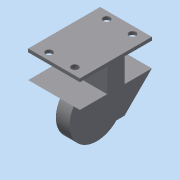
# Autodesk Inventor part: caster wheel
Saved by Autodesk Inventor 2015 (Build 190159000, 159)
## iProperties
Created: 2015-06-24
Part Number: caster wheel
Material: Generic
Document SubType Name: Modeling
Designer: Rahul
Density: 1 g/cm^3
Appearance: Default
Author: Rahul
Autodesk Inventor part; units mm, degrees
ref_plane "YZ Plane" through (0, 0, 0) normal (1, 0, 0) x (0, 1, 0)
ref_plane "XZ Plane" through (0, 0, 0) normal (0, 1, 0) x (-1, 0, 0)
ref_plane "XY Plane" through (0, 0, 0) normal (0, 0, 1) x (1, 0, 0)
sketch "Sketch10" plane through (0, 0, 0) normal (0, 1, 0) x (-1, 0, 0)
  line L0 (24.0538, -33.4645) -> (-24.0538, -33.4645)
  line L1 (-24.0538, -33.4645) -> (-24.0538, 33.4645)
  line L2 (-24.0538, 33.4645) -> (24.0538, 33.4645)
  line L3 (24.0538, 33.4645) -> (24.0538, -33.4645)
  line L4 (33.6753, 0) -> (-33.6753, 0) projected
  line L5 (0, -46.8503) -> (0, 46.8503) projected
  point P0 (0, 0)
  dimension "d17" = 66.929
  dimension "d18" = 48.1076
  constraints: 8 end point, 2 parallel, 1 horizontal, 1 perpendicular, 2 other
  measures "d17" distance of L0.end L1.end
  measures "d18" distance of L0.start L0.end
extrude "Extrusion4" add sketch "Sketch10" against normal blind 50.8
sketch "Sketch11" plane through (0, -50.8, 0) normal (0, -1, 0) x (1, 0, 0)
  line L0 (6.35, 25.4) -> (-6.35, 25.4)
  line L1 (-6.35, 25.4) -> (-6.35, 0)
  line L2 (-6.35, 0) -> (6.35, 0)
  line L3 (6.35, 0) -> (6.35, 25.4)
  line L4 (-33.6753, 0) -> (33.6753, 0) projected
  line L5 (0, -46.8503) -> (0, 46.8503) projected
  point P0 (0, 0)
  dimension "d21" = 25.4
  dimension "d22" = 12.7
  constraints: 8 end point, 2 parallel, 1 collinear, 1 horizontal, 1 perpendicular, 1 other
  measures "d21" distance of L2.end L0.start
  measures "d22" distance of L1.end L2.end
revolve "Revolution3" add sketch "Sketch11" angle 360 about axis through (-6.35, -50.8, 0) along (1, 0, 0)
chamfer "Chamfer2" distance 25.4 angle 45 2 edges at (0, -50.8, -33.4645) (0, -50.8, 33.4645)
sketch "Sketch12" plane through (0, 0, 0) normal (0, 1, 0) x (1, 0, 0)
  circle A0 centre (12.7508, 26.7462) radius 3.2195
  line L0 (-24.0538, 33.4645) -> (24.0538, 33.4645) projected
  line L1 (24.0538, 33.4645) -> (24.0538, 8.0645) projected
  circle A1 centre (-11.2649, 26.7462) radius 3.2195
  circle A2 centre (12.7508, -26.8097) radius 3.2195
  circle A3 centre (-11.2649, -26.8097) radius 3.2195
  point P0 (0, 0)
  dimension "d27" = 6.4389
  dimension "d28" = 6.7183
  dimension "d29" = 11.303
  dimension "d32" = 24.0157
  dimension "d42" = 53.5559
  dimension "d46" = 24.0157
  constraints: 4 centre point, 2 horizontal, 1 vertical, 6 other
  measures "d27" diameter of A0
  measures "d28" distance from line of L0 A0.centre
  measures "d29" distance from line of L1 A0.centre
  measures "d32" distance of A0.centre A1.centre
  measures "d42" distance of A0.centre A2.centre
  measures "d46" distance of A2.centre A3.centre
extrude "Extrusion5" cut sketch "Sketch12" against normal blind 5.08
sketch "Sketch13" plane through (-24.0538, 0, 33.4645) normal (0, 0, 1) x (1, 0, 0)
  line L0 (0, 0) -> (0, -25.4) projected
  line L1 (0, -3.0578) -> (48.1076, -3.0578)
  line L2 (48.1076, -3.0578) -> (48.1076, -25.4)
  line L3 (48.1076, -25.4) -> (0, -25.4)
  line L4 (0, -25.4) -> (0, -3.0578)
  constraints: 8 end point, 2 parallel, 1 horizontal, 1 perpendicular, 1 point on line
extrude "Extrusion6" cut sketch "Sketch13" against normal blind 25.4
sketch "Sketch14" plane through (24.0538, 0, -33.4645) normal (0, 0, -1) x (-1, 0, 0)
  line L0 (0, -3.0578) -> (48.1076, -3.0578)
  line L1 (48.1076, -3.0578) -> (48.1076, -25.4)
  line L2 (48.1076, -25.4) -> (0, -25.4)
  line L3 (0, -25.4) -> (0, -3.0578)
  point P0 (24.0538, 0)
  constraints: 8 end point, 2 parallel, 1 horizontal, 1 perpendicular
extrude "Extrusion7" cut sketch "Sketch14" against normal blind 25.4
body "Solid2"
